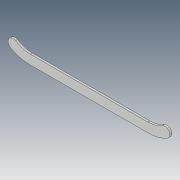
# Autodesk Inventor part: bottomSkid
Saved by Autodesk Inventor 2018 (Build 220112000, 112)
## iProperties
Created: 2020-02-18
Part Number: bottomSkid
Material: Generic
Document SubType Name: Modeling
Designer: anirudh
Density: 1 g/cm^3
Appearance: Default
Author: anirudh
Autodesk Inventor part; units mm, degrees
ref_plane "YZ Plane" through (0, 0, 0) normal (1, 0, 0) x (0, 1, 0)
ref_plane "XZ Plane" through (0, 0, 0) normal (0, 1, 0) x (-1, 0, 0)
ref_plane "XY Plane" through (0, 0, 0) normal (0, 0, 1) x (1, 0, 0)
sketch "Sketch1" plane through (0, 0, 0) normal (0, 0, 1) x (1, 0, 0)
  line L0 (55.4931, -0.0207) -> (359.029, -0.0207)
  line L1 (208.28, -0.0207) -> (55.4931, -0.0207)
  line L2 (208.28, -0.0207) -> (359.029, -0.0207)
  line L3 (57.245, 23.9209) -> (359.029, 23.9209)
  line L4 (208.28, -0.0207) -> (359.029, -0.0207)
  line L5 (55.4931, -0.0207) -> (359.0367, -0.0207)
  line L6 (359.0367, 23.9209) -> (57.245, 23.9209)
  arc A0 (19.6495, 34.5513) -> (6.6543, 12.7528) centre (12.7, 23.9214) ccw
  arc A1 (19.138, 34.8687) -> (57.245, 23.9209) centre (57.245, 95.7161) ccw
  arc A2 (6.262, 12.9742) -> (55.4931, -0.0207) centre (55.4931, 99.7327) ccw
  arc A3 (409.6274, 12.7528) -> (396.6322, 34.5513) centre (403.5817, 23.9214) ccw
  arc A4 (359.0367, 23.9209) -> (397.1436, 34.8687) centre (359.0367, 95.7161) ccw
  arc A5 (360.7886, -0.0207) -> (410.0197, 12.9742) centre (360.7886, 99.7327) ccw
  line L7 (360.7886, -0.0207) -> (55.4931, -0.0207)
  point P0 (0, 0)
  point P1 (416.2817, 0)
  constraints: 20 point on circle, 16 end point, 6 centre point, 3 horizontal, 3 tangent, 2 collinear, 1 point on line
extrude "Extrusion1" add sketch "Sketch1" along normal blind 5.08 contours A2 A0 A1 L3 L6 A4 A3 A5 L7 L5 L0
body "Solid1"
